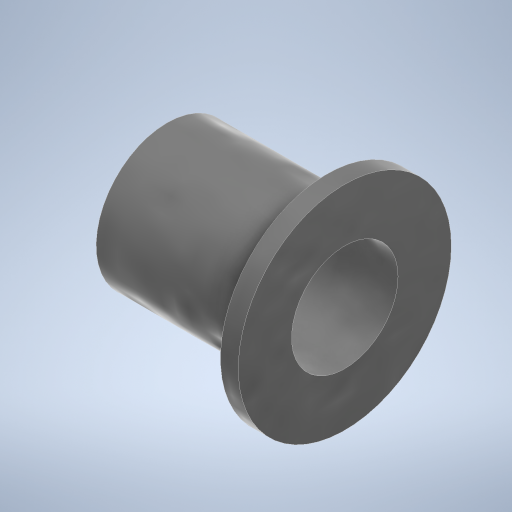
# Autodesk Inventor part: oiles_bush6-10
Saved by Autodesk Inventor 2024.1 (Build 281209000, 209)
## iProperties
Created: 2023-10-03
Part Number: oiles_bush6-10
Material: ABS プラスチック
Document SubType Name: Modeling
Designer: haruy
Density: 1.06 g/cm^3
Appearance: 細かい テクスチャ - 黒
Author: haruy
Autodesk Inventor part; units mm, degrees
ref_plane "YZ Plane" through (0, 0, 0) normal (1, 0, 0) x (0, 1, 0)
ref_plane "XZ Plane" through (0, 0, 0) normal (0, 1, 0) x (-1, 0, 0)
ref_plane "XY Plane" through (0, 0, 0) normal (0, 0, 1) x (1, 0, 0)
sketch "スケッチ1" plane through (0, 0, 0) normal (1, 0, 0) x (0, 1, 0)
  circle A0 centre (0, 0) radius 3
  circle A1 centre (0, 0) radius 4
  dimension "d0" = 6
  dimension "d1" = 8
  constraints: 2 centre point, 2 coincident
  measures "d0" diameter of A0
  measures "d1" diameter of A1
extrude "押し出し1" add sketch "スケッチ1" along normal blind 9
sketch "スケッチ2" plane through (9, 0, 0) normal (1, 0, 0) x (0, 0, -1)
  circle A0 centre (0, 0) radius 6
  circle A1 centre (0, 0) radius 3
  dimension "d4" = 12
  constraints: 2 centre point, 2 coincident
  measures "d4" diameter of A0
extrude "押し出し2" add sketch "スケッチ2" along normal blind 1
